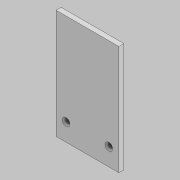
# Autodesk Inventor part: cover
Saved by Autodesk Inventor 2021.4 (Build 254397000, 397)
## iProperties
Created: 2022-11-07
Part Number: cover
Material: Generisch
Document SubType Name: Modeling
Designer: Tilman Preuschoff
Density: 1 g/cm^3
Appearance: Vorgabe
Author: Tilman Preuschoff
Autodesk Inventor part; units mm, degrees
ref_plane "YZ Plane" through (0, 0, 0) normal (1, 0, 0) x (0, 1, 0)
ref_plane "XZ Plane" through (0, 0, 0) normal (0, 1, 0) x (-1, 0, 0)
ref_plane "XY Plane" through (0, 0, 0) normal (0, 0, 1) x (1, 0, 0)
sketch "Skizze1" plane through (0, 0, 0) normal (0, 0, 1) x (1, 0, 0)
  line L0 (-12.5, 21.75) -> (12.5, 21.75)
  line L1 (12.5, 21.75) -> (12.5, -21.75)
  line L2 (12.5, -21.75) -> (-12.5, -21.75)
  line L3 (-12.5, -21.75) -> (-12.5, 21.75)
  line L4 (-12.5, 21.75) -> (12.5, -21.75) construction
  line L5 (12.5, 21.75) -> (-12.5, -21.75) construction
  point P0 (0, 0)
  dimension "d0" = 25
  dimension "d1" = 43.5
  constraints: 12 end point, 2 midpoint, 2 parallel, 1 horizontal, 1 perpendicular
  measures "d0" distance between parallel lines of L1 L3
  measures "d1" distance between parallel lines of L2 L0
extrude "Extrusion1" add sketch "Skizze1" along normal blind 2
sketch "Skizze2" plane through (0, 0, 2) normal (0, 0, 1) x (1, 0, 0)
  line L0 (12.5, 21.75) -> (-12.5, 21.75) projected
  line L1 (-12.5, 21.75) -> (-12.5, -21.75) projected
  line L2 (-12.5, -21.75) -> (12.5, -21.75) projected
  line L3 (12.5, -21.75) -> (12.5, 21.75) projected
  point P0 (0, 0)
  point P1 (-8.5, -14.75)
  point P2 (8.5, -14.75)
  dimension "d5" = 4
  dimension "d6" = 7
  dimension "d7" = 4
  dimension "d15" = 7
  measures "d5" distance from line of L1 point (-8.5, -14.75)
  measures "d6" distance from line of L2 point (8.5, -14.75)
  measures "d7" distance from line of L3 point (8.5, -14.75)
  measures "d15" distance from line of L2 point (-8.5, -14.75)
hole "Bohrung1" at (-8.5, -14.75, 2) at (8.5, -14.75, 2) direction (0, 0, -1) diameter 1.778 end through all countersink diameter 3.023 countersink angle 82 clearance for "Flachkopfmaschinenschraube (82)" size "#0" standard "ANSI UST"
